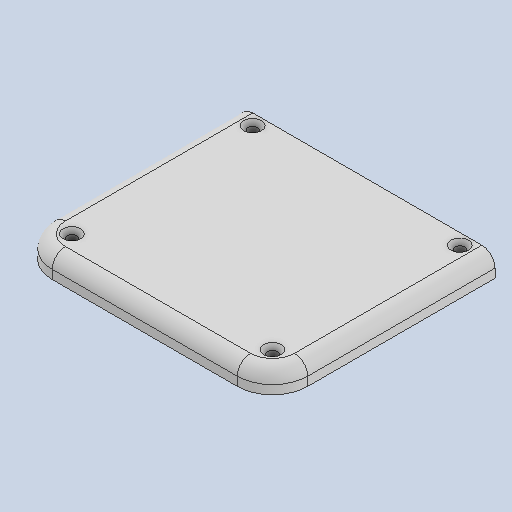
# Autodesk Inventor part: Closing_Stepper_2
Saved by Autodesk Inventor 2022.3 (Build 263350000, 350)
## iProperties
Created: 2023-03-29
Part Number: Closing_Stepper_2
Material: Generic
Document SubType Name: Modeling
Designer: Manuel Hueso Béjar
Density: 1 g/cm^3
Appearance: Default
Author: Manuel Hueso Béjar
Autodesk Inventor part; units mm, degrees
ref_plane "YZ Plane" through (0, 0, 0) normal (1, 0, 0) x (0, 1, 0)
ref_plane "XZ Plane" through (0, 0, 0) normal (0, 1, 0) x (-1, 0, 0)
ref_plane "XY Plane" through (0, 0, 0) normal (0, 0, 1) x (1, 0, 0)
sketch "Sketch1" plane through (0, 0, 0) normal (0, 1, 0) x (-1, 0, 0)
  line L0 (-26, 23.75) -> (26, 23.75)
  line L1 (26, 23.75) -> (26, -23.75)
  line L2 (26, -23.75) -> (-26, -23.75)
  line L3 (-26, -23.75) -> (-26, 23.75)
  line L4 (-26, 23.75) -> (26, -23.75) construction
  line L5 (26, 23.75) -> (-26, -23.75) construction
  point P0 (0, 0)
  dimension "d0" = 52
  dimension "d1" = 47.5
  constraints: 12 end point, 2 midpoint, 2 parallel, 1 horizontal, 1 perpendicular
  measures "d0" distance of L1.end L2.end
  measures "d1" distance of L0.end L1.end
extrude "Extrusion1" add sketch "Sketch1" along normal blind 3
fillet "Fillet1" radius 5 2 edges at (26, 1.5, 23.75) (-26, 1.5, 23.75)
sketch "Sketch2" plane through (0, 3, 0) normal (0, 1, 0) x (1, 0, 0)
  arc A0 (-26, -18.75) -> (-21, -23.75) centre (-21, -18.75) ccw projected
  line L0 (-21, -23.75) -> (21, -23.75) projected
  arc A1 (21, -23.75) -> (26, -18.75) centre (21, -18.75) ccw projected
  line L1 (26, -18.75) -> (26, 23.75) projected
  line L2 (26, 23.75) -> (-26, 23.75) projected
  line L3 (-26, 23.75) -> (-26, -18.75) projected
  line L4 (29, 26.75) -> (29, -18.75)
  arc A2 (21, -26.75) -> (29, -18.75) centre (21, -18.75) ccw
  line L5 (21, -26.75) -> (-21, -26.75)
  arc A3 (-29, -18.75) -> (-21, -26.75) centre (-21, -18.75) ccw
  line L6 (-29, -18.75) -> (-29, 26.75)
  line L7 (-29, 26.75) -> (29, 26.75)
  point P0 (0, 0)
  dimension "d5" = 3
  constraints: 8 end point, 4 point on circle, 2 centre point, 5 other
  measures "d5" distance between parallel lines of L1 L4
extrude "Extrusion2" add sketch "Sketch2" against normal blind 5
sketch "Sketch3" plane through (0, 3, 0) normal (0, 1, 0) x (1, 0, 0)
  line L0 (26, -18.75) -> (26, 23.75) projected
  line L1 (29, 26.75) -> (26, 26.75)
  line L2 (26, 26.75) -> (26, 23.75)
  line L3 (26, 23.75) -> (29, 23.75)
  line L4 (29, 23.75) -> (29, 26.75)
  line L5 (26, 23.75) -> (21, 23.75)
  line L6 (21, 23.75) -> (21, 18.75)
  line L7 (21, 18.75) -> (26, 18.75)
  line L8 (26, 18.75) -> (26, 23.75)
  line L9 (-29, 26.75) -> (-26, 26.75)
  line L10 (-26, 26.75) -> (-26, 23.75)
  line L11 (-26, 23.75) -> (-29, 23.75)
  line L12 (-29, 23.75) -> (-29, 26.75)
  line L13 (-26, 23.75) -> (-21, 23.75)
  line L14 (-21, 23.75) -> (-21, 18.75)
  line L15 (-21, 18.75) -> (-26, 18.75)
  line L16 (-26, 18.75) -> (-26, 23.75)
  arc A0 (-29, -18.75) -> (-21, -26.75) centre (-21, -18.75) ccw projected
  line L17 (21, 18.75) -> (-21, 18.75)
  line L18 (-21, 18.75) -> (-21, -18.75)
  line L19 (-21, -18.75) -> (21, -18.75)
  line L20 (21, -18.75) -> (21, 18.75)
  line L21 (-21, -18.75) -> (-26, -18.75)
  line L22 (-26, -18.75) -> (-26, -23.75)
  line L23 (-26, -23.75) -> (-21, -23.75)
  line L24 (-21, -23.75) -> (-21, -18.75)
  line L25 (-21, -18.75) -> (-24.5355, -22.2855)
  line L26 (-21, -18.75) -> (-16, -18.75) construction
  line L27 (21, -18.75) -> (24.5355, -22.2855)
  line L28 (24.5355, -22.2855) -> (-24.5355, -22.2855)
  line L29 (26, 18.75) -> (21, 23.75)
  line L30 (-21, 23.75) -> (-26, 18.75)
  line L31 (22.7678, -20.5178) -> (-22.7678, -20.5178)
  line L32 (23.5, 21.25) -> (-23.5, 21.25)
  point P0 (0, 0)
  dimension "d8" = 3
  dimension "d9" = 3
  dimension "d10" = 5
  dimension "d11" = 5
  dimension "d12" = 3
  dimension "d13" = 3
  dimension "d14" = 5
  dimension "d15" = 5
  dimension "d16" = 37.5
  dimension "d17" = 5
  dimension "d18" = 5
  dimension "d19" = 5
  dimension "d20" = 135
  dimension "d21" = 5
  constraints: 64 end point, 12 parallel, 8 horizontal, 6 perpendicular, 4 midpoint, 1 equal length
  measures "d8" distance of L3.end L0.end
  measures "d9" distance of L0.end L1.end
  measures "d10" distance of L7.end L6.end
  measures "d11" distance of L6.end L5.end
  measures "d12" distance of L10.end L11.end
  measures "d13" distance of L9.end L10.end
  measures "d14" distance of L14.end L15.end
  measures "d15" distance of L13.end L14.end
  measures "d16" distance of L18.end L17.end
  measures "d17" distance of L23.end L22.end
  measures "d18" distance of L22.end L21.end
  measures "d19" distance of L18.end L25.end
  measures "d20" angle of L25 L26
  measures "d21" distance of L19.end L27.end
hole "Hole1" at (-23.5, 3, -21.25) at (23.5, 3, -21.25) at (22.7678, 3, 20.5178) at (-22.7678, 3, 20.5178) direction (0, -1, 0) diameter 2.2 end through all countersink diameter 4 countersink angle 90
fillet "Fillet2" radius 3 5 edges at (26.6569, 3, 24.4069) (0, 3, 26.75) (-26.6569, 3, 24.4069) (-29, 3, -4) (29, 3, -4)
thicken "Thicken1" operation add thickness 3 both sides no extend neighbours yes toward (0, 0, 1) faces at (8.6667, -0.3333, -26.75)
body "Solid1"
